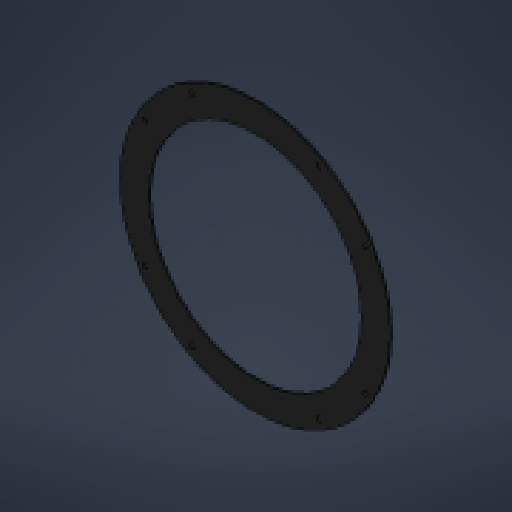
# Autodesk Inventor part: 3DPRINT,TURRET,SPACER
Saved by Autodesk Inventor 2026.1 (Build 301233020, 233B)
## iProperties
Created: 2026-02-09
Part Number: 3DPRINT,TURRET,SPACER
Material: Nylon 6/6
Document SubType Name: Modeling
Designer: littl
Density: 1.13 g/cm^3
Appearance: Smooth - Black
Author: littl
Autodesk Inventor part; units mm, degrees
ref_plane "YZ Plane" through (0, 0, 0) normal (1, 0, 0) x (0, 1, 0)
ref_plane "XZ Plane" through (0, 0, 0) normal (0, 1, 0) x (-1, 0, 0)
ref_plane "XY Plane" through (0, 0, 0) normal (0, 0, 1) x (1, 0, 0)
sketch "Sketch1" plane through (0, 0, 0) normal (0, 0, 1) x (1, 0, 0)
  circle A0 centre (0, 0) radius 106.3625
  circle A1 centre (0, 0) radius 134.9375
  dimension "d0" = 212.725
  dimension "d1" = 269.875
  constraints: 2 centre point, 2 coincident
  measures "d0" diameter of A0
  measures "d1" diameter of A1
extrude "Extrusion1" add sketch "Sketch1" along normal blind 1.5875
sketch "Sketch2" plane through (0, 0, 1.5875) normal (0, 0, 1) x (1, 0, 0)
  point P0 (0, 0)
  point P1 (0, 127)
  point P2 (-63.5, 109.9852)
  point P3 (-109.9852, 63.5)
  point P4 (-127, 0)
  point P5 (-109.9852, -63.5)
  point P6 (-63.5, -109.9852)
  point P7 (0, -127)
  point P8 (63.5, -109.9852)
  point P9 (109.9852, -63.5)
  point P10 (127, 0)
  point P11 (109.9852, 63.5)
  point P12 (63.5, 109.9852)
  dimension "d4" = 127
  dimension "d7" = 360
  constraints: 1 vertical alignment, 13 other
  measures "d4" distance of point (0, 0) point (0, 127)
hole "Hole1" at (-63.5, 109.9852, 1.5875) at (-109.9852, 63.5, 1.5875) at (-109.9852, -63.5, 1.5875) at (-63.5, -109.9852, 1.5875) at (63.5, 109.9852, 1.5875) at (109.9852, 63.5, 1.5875) at (109.9852, -63.5, 1.5875) at (63.5, -109.9852, 1.5875) direction (0, 0, -1) diameter 4.9784 end through all clearance for "Flat Head Machine Screw (82)" size "#10" standard "Ansi Unified Screw Threads"
body "Solid1"
